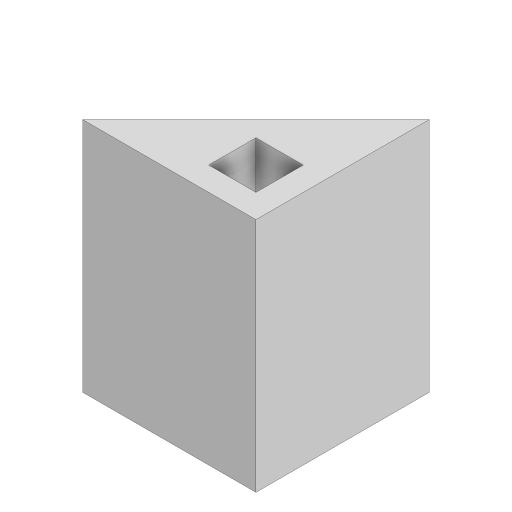
# Autodesk Inventor part: triangle
Saved by Autodesk Inventor 2024 (Build 280153000, 153)
## iProperties
Created: 2024-05-23
Part Number: triangle
Material: 一般
Document SubType Name: Modeling
Designer: USER
Density: 1 g/cm^3
Appearance: 預設
Author: USER
Autodesk Inventor part; units mm, degrees
ref_plane "YZ Plane" through (0, 0, 0) normal (1, 0, 0) x (0, 1, 0)
ref_plane "XZ Plane" through (0, 0, 0) normal (0, 1, 0) x (-1, 0, 0)
ref_plane "XY Plane" through (0, 0, 0) normal (0, 0, 1) x (1, 0, 0)
sketch "草圖1" plane through (0, 0, 0) normal (0, 1, 0) x (-1, 0, 0)
  line L0 (0, 0) -> (0, -11)
  line L1 (0, -11) -> (11, 0)
  line L2 (11, 0) -> (0, 0)
  line L3 (4.5, -1.5) -> (1.5, -1.5)
  line L4 (1.5, -1.5) -> (1.5, -4.5)
  line L5 (1.5, -4.5) -> (4.5, -4.5)
  line L6 (4.5, -4.5) -> (4.5, -1.5)
  dimension "d0" = 11
  dimension "d1" = 11
  dimension "d4" = 3
  dimension "d5" = 3
  dimension "d8" = 1.5
  dimension "d9" = 1.5
  constraints: 14 end point, 2 parallel, 2 perpendicular, 1 horizontal, 1 vertical
  measures "d0" distance of L0.start L0.end
  measures "d1" distance of L1.end L0.start
  measures "d4" distance of L3.end L4.end
  measures "d5" distance of L4.end L5.end
  measures "d8" horizontal distance of L0.start L3.end
  measures "d9" horizontal distance of L0.start L3.end
extrude "擠出1" add sketch "草圖1" along normal blind 15
